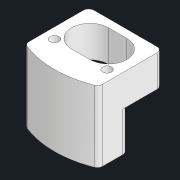
# Autodesk Inventor part: scara-base13
Saved by Autodesk Inventor 2022 (Build 260153000, 153)
## iProperties
Created: 2021-10-28
Part Number: scara-base13
Material: ABS プラスチック
Document SubType Name: Modeling
Designer: Yuta Kage
Density: 1.06 g/cm^3
Appearance: 滑らか - 白
Author: Yuta Kage
Autodesk Inventor part; units mm, degrees
ref_plane "YZ Plane" through (0, 0, 0) normal (1, 0, 0) x (0, 1, 0)
ref_plane "XZ Plane" through (0, 0, 0) normal (0, 1, 0) x (-1, 0, 0)
ref_plane "XY Plane" through (0, 0, 0) normal (0, 0, 1) x (1, 0, 0)
sketch "スケッチ1" plane through (0, 0, 0) normal (0, 1, 0) x (-1, 0, 0)
  circle A0 centre (0, 0) radius 34.996
  circle A1 centre (0, 18) radius 10
  line L0 (48.9944, 0) -> (-48.9944, 0) projected
  line L1 (-14, 8) -> (14, 8)
  line L2 (14, 8) -> (14, 32.0737)
  line L3 (14, 32.0737) -> (-14, 32.0737)
  line L4 (-14, 32.0737) -> (-14, 8)
  line L5 (-14, 8) -> (14, 32.0737) construction
  line L6 (14, 8) -> (-14, 32.0737) construction
  point P0 (10, 25)
  point P1 (-10, 25)
  point P2 (0, 20.0368)
  dimension "d0" = 25
  dimension "d1" = 10
  dimension "d2" = 10
  dimension "d3" = 69.992
  dimension "d5" = 20
  dimension "d7" = 18
  dimension "d8" = 4
  constraints: 12 end point, 2 centre point, 2 midpoint, 2 parallel, 2 point on circle, 1 coincident, 1 horizontal, 1 horizontal alignment, 1 perpendicular, 1 tangent, 1 vertical alignment
  measures "d0" vertical distance of point (0, 0) point (10, 25)
  measures "d1" horizontal distance of point (0, 0) point (10, 25)
  measures "d2" horizontal distance of point (-10, 25) point (0, 0)
  measures "d3" diameter of A0
  measures "d5" diameter of A1
  measures "d7" distance from line of L0 A1.centre
  measures "d8" distance from line of L2 point (10, 25)
extrude "押し出し1" add sketch "スケッチ1" along normal blind 27 contours L3 A0 | A1 | L2 L1 L4 L3
hole "穴1" at (-10, 0, 25) at (10, 0, 25) direction (0, 1, 0) diameter 3.4 end through all clearance for "Flat Head Machine Screw" size "M3" standard "Ansi Metric M Profile"
sketch "スケッチ2" plane through (0, 0, 0) normal (0, -1, 0) x (1, 0, 0)
  circle A0 centre (3.5, 18) radius 7 construction
  circle A1 centre (-7, 18) radius 3.5 construction
  line L0 (-3.5, 18) -> (3.5, 18) construction
  line L1 (-3.5, 11) -> (3.5, 11)
  line L2 (3.5, 25) -> (-3.5, 25)
  arc A2 (-3.5, 25) -> (-3.5, 11) centre (-3.5, 18) ccw
  arc A3 (3.5, 11) -> (3.5, 25) centre (3.5, 18) ccw
  point P0 (0, 0)
  point P1 (0, 18)
  point P2 (-10.5, 18)
  dimension "d31" = 7
  dimension "d30" = 14
  dimension "d32" = 7
  constraints: 8 end point, 5 point on circle, 4 tangent, 3 centre point, 3 horizontal alignment, 1 concentric, 1 horizontal, 1 midpoint, 1 parallel, 3 other
  measures "d30" diameter of A0
  measures "d32" radius of A3
extrude "押し出し2" cut sketch "スケッチ2" against normal through all
sketch "スケッチ3" plane through (0, 0, 0) normal (0, -1, 0) x (1, 0, 0)
  line L0 (14, 8) -> (-14, 8) projected
  line L1 (14, -21) -> (-14, -21)
  line L2 (-14, -21) -> (-14, 21)
  line L3 (-14, 21) -> (14, 21)
  line L4 (14, 21) -> (14, -21)
  line L5 (14, -21) -> (-14, 21) construction
  line L6 (-14, -21) -> (14, 21) construction
  circle A0 centre (-10, 25) radius 1.7 projected
  point P0 (0, 0)
  point P1 (-14, 8)
  dimension "d25" = 4
  constraints: 12 end point, 2 midpoint, 2 parallel, 1 horizontal, 1 perpendicular, 1 point on line
  measures "d25" distance from line of L3 A0.centre
extrude "押し出し3" cut sketch "スケッチ3" against normal blind 15 contours L0 L2 L3 L4
fillet "フィレット2" radius 2 8 edges at (14, 21, 8) (14, 7.5, 21) (-14, 7.5, 21) (-14, 21, 8) (14, 13.5, 32.0737) (-14, 13.5, 32.0737) (9.8246, 7.5, 21) (-9.8246, 7.5, 21)
equation "\"d2\" = d1"
equation "\"d32\" = 0.5 * d30"
